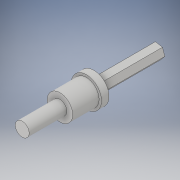
# Autodesk Inventor part: Shaft
Saved by Autodesk Inventor 2018 (Build 220112000, 112)
## iProperties
Created: 2018-04-27
Part Number: Shaft
Material: Generic
Document SubType Name: Modeling
Designer: Samuel
Density: 1 g/cm^3
Appearance: Default
Author: Samuel
## iProperties of the stored document Shaft_3DPrint.ipt
Created: 2018-04-27
Part Number: Shaft_3DPrint
Material: Generic
Document SubType Name: Modeling
Designer: Samuel
Density: 1 g/cm^3
Appearance: Default
Author: Samuel
Autodesk Inventor part; units mm, degrees
ref_plane "YZ Plane" through (0, 0, 0) normal (1, 0, 0) x (0, 1, 0)
ref_plane "XZ Plane" through (0, 0, 0) normal (0, 1, 0) x (-1, 0, 0)
ref_plane "XY Plane" through (0, 0, 0) normal (0, 0, 1) x (1, 0, 0)
sketch "Sketch1" plane through (0, 0, 0) normal (0, 0, 1) x (1, 0, 0)
  circle A0 centre (0, 0) radius 4.5 construction
  line L0 (-1.8766, -2.1935) -> (-2.838, 0.5284) construction
  line L1 (-2.838, 0.5284) -> (-0.9614, 2.722) construction
  line L2 (-0.9614, 2.722) -> (1.8766, 2.1935) construction
  line L3 (1.8766, 2.1935) -> (2.838, -0.5284) construction
  line L4 (2.838, -0.5284) -> (0.9614, -2.722) construction
  line L5 (0.9614, -2.722) -> (-1.8766, -2.1935) construction
  line L6 (-0.9498, 2.6893) -> (-2.8039, 0.5221)
  line L7 (-2.8039, 0.5221) -> (-1.8541, -2.1672)
  line L8 (-1.8541, -2.1672) -> (0.9498, -2.6893)
  line L9 (0.9498, -2.6893) -> (2.8039, -0.5221)
  line L10 (2.8039, -0.5221) -> (1.8541, 2.1672)
  line L11 (1.8541, 2.1672) -> (-0.9498, 2.6893)
  dimension "d0" = 0.03
  constraints: 12 end point, 5 other
  measures "d0" distance between parallel lines of L1 L6
extrude "Extrusion1" add sketch "Sketch1" against normal blind 25.4
sketch "Sketch2" plane through (0, 0, 0) normal (0, 0, 1) x (1, 0, 0)
  circle A0 centre (0, 0) radius 6
  dimension "d3" = 12
  constraints: 1 centre point, 1 coincident
  measures "d3" diameter of A0
extrude "Extrusion2" add sketch "Sketch2" along normal blind 3
sketch "Sketch4" plane through (0, 0, 3) normal (0, 0, 1) x (1, 0, 0)
  circle A0 centre (0, 0) radius 5.08 construction
  circle A1 centre (0, 8) radius 1.48 construction
  circle A2 centre (6.9282, 4) radius 1.48 construction
  circle A3 centre (6.9282, -4) radius 1.48 construction
  circle A4 centre (0, -8) radius 1.48 construction
  circle A5 centre (-6.9282, -4) radius 1.48 construction
  circle A6 centre (-6.9282, 4) radius 1.48 construction
  circle A7 centre (0, 0) radius 5.05
  circle A8 centre (0, 0) radius 12.7 projected
  point P0 (0, 0)
  dimension "d7" = 0.03
  constraints: 1 centre point
  measures "d7" radial gap between concentric circles of A0 A7
extrude "Extrusion3" add sketch "Sketch4" along normal blind 10.5 contours A7
sketch "Sketch5" plane through (0, 0, 13.5) normal (0, 0, 1) x (1, 0, 0)
  circle A0 centre (0, 0) radius 2.75
  point P0 (0, 0)
  dimension "d10" = 5.5
  constraints: 1 centre point, 1 coincident
  measures "d10" diameter of A0
extrude "Extrusion4" add sketch "Sketch5" along normal blind 15
body "Solid1"
